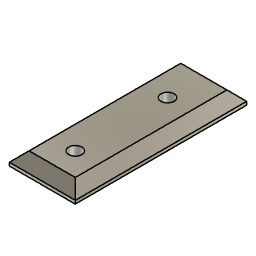
screw_mount v1 (Autodesk Fusion 360 design; units mm, degrees)
Autodesk Fusion 360 part; units mm, degrees
sketch "Sketch1" plane through (0, 0, 0) normal (0, 0, 1) x (1, 0, 0)
  line L0 (0, 0) -> (-10, 0)
  line L1 (-10, 0) -> (-10, -26)
  line L2 (-10, -26) -> (0, -26)
  line L3 (0, -26) -> (0, 0)
  dimension "d1" = 10
  dimension "d2" = 26
  constraint horizontal L0
  constraint vertical L1
  constraint horizontal L2
  constraint vertical L3
  constraint coincident L0.start L3.end
  measures "d1" distance of L0.start L0.end
  measures "d2" distance of L0.start L2.end
extrude "Extrude1" add sketch "Sketch1" along normal blind 2
sketch "Sketch2" plane through (0, 0, 2) normal (0, 0, 1) x (-1, 0, 0)
  line L0 (0, 26) -> (0, 0)
  line L1 (0, 0) -> (10, 0)
  line L2 (10, 0) -> (10, 26)
  line L3 (10, 26) -> (0, 26)
  circle A0 centre (5, 21) radius 1
  circle A1 centre (5, 7.0039) radius 1
  point P0 (4.5847, 3.0102)
  dimension "d5" = 2
  dimension "d6" = 2
  dimension "d8" = 5
  dimension "d9" = 5
  dimension "d10" = 13.9961
  dimension "d11" = 5
  measures "d5" diameter of A0
  measures "d6" diameter of A1
  measures "d8" distance of L2 A0.centre
  measures "d9" distance of L2 A1.centre
  measures "d10" distance of A0.centre A1.centre
  measures "d11" distance of L3 A0.centre
extrude "Extrude2" cut sketch "Sketch2" against normal blind 10 contours A0 | A1
chamfer "Chamfer1" distance 1.5 angle 45 4 edges at (-5, -26, 2) (0, -13, 2) (-10, -13, 2) (-5, 0, 2) measured on face at (-5.0249, -2.0022, 2) measured on face at (-5.0249, -2.0022, 2) measured on face at (-5.0249, -2.0022, 2) measured on face at (-5.0249, -2.0022, 2)
